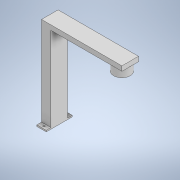
# Autodesk Inventor part: main_stand_upper_half
Saved by Autodesk Inventor 2021 (Build 250183000, 183)
## iProperties
Created: 2020-10-10
Part Number: main_stand_upper_half
Material: Generic
Document SubType Name: Modeling
Designer: bober
Density: 1 g/cm^3
Appearance: Default
Author: bober
Autodesk Inventor part; units mm, degrees
ref_plane "YZ Plane" through (0, 0, 0) normal (1, 0, 0) x (0, 1, 0)
ref_plane "XZ Plane" through (0, 0, 0) normal (0, 1, 0) x (-1, 0, 0)
ref_plane "XY Plane" through (0, 0, 0) normal (0, 0, 1) x (1, 0, 0)
sketch "Sketch1" plane through (0, 0, 0) normal (0, 1, 0) x (-1, 0, 0)
  line L0 (-10, 27.5) -> (10, 27.5)
  line L1 (10, 27.5) -> (10, -27.5)
  line L2 (10, -27.5) -> (-10, -27.5)
  line L3 (-10, -27.5) -> (-10, 27.5)
  line L4 (-10, 27.5) -> (10, -27.5) construction
  line L5 (10, 27.5) -> (-10, -27.5) construction
  point P0 (0, 0)
  dimension "d0" = 20
  dimension "d1" = 55
  constraints: 12 end point, 2 midpoint, 2 parallel, 1 horizontal, 1 perpendicular
  measures "d0" distance of L1.end L2.end
  measures "d1" distance of L0.end L1.end
extrude "Extrusion1" add sketch "Sketch1" along normal blind 3
sketch "Sketch2" plane through (0, 3, 0) normal (0, 1, 0) x (1, 0, 0)
  circle A0 centre (0, -22.5) radius 2
  circle A1 centre (0, 22.5) radius 2
  point P0 (0, 0)
  dimension "d4" = 4
  dimension "d5" = 4
  constraints: 2 centre point
  measures "d4" diameter of A0
  measures "d5" diameter of A1
extrude "Extrusion2" cut sketch "Sketch2" against normal blind 3
sketch "Sketch3" plane through (0, 3, 0) normal (0, 1, 0) x (1, 0, 0)
  line L0 (10, -17.5) -> (-10, -17.5)
  line L1 (-10, -17.5) -> (-10, 17.5)
  line L2 (-10, 17.5) -> (10, 17.5)
  line L3 (10, 17.5) -> (10, -17.5)
  line L4 (10, -17.5) -> (-10, 17.5) construction
  line L5 (-10, -17.5) -> (10, 17.5) construction
  point P0 (0, 0)
  dimension "d8" = 20
  dimension "d9" = 35
  constraints: 12 end point, 2 midpoint, 2 parallel, 1 horizontal, 1 perpendicular
  measures "d8" distance of L1.end L2.end
  measures "d9" distance of L0.end L1.end
extrude "Extrusion3" add sketch "Sketch3" along normal blind 178
sketch "Sketch4" plane through (0, 181, 0) normal (0, 1, 0) x (1, 0, 0)
  line L0 (-10, 17.5) -> (-10, -17.5) projected
  line L1 (-10, -17.5) -> (160, -17.5)
  line L2 (160, -17.5) -> (160, 17.5)
  line L3 (160, 17.5) -> (-10, 17.5)
  line L4 (-10, 17.5) -> (-10, -17.5)
  point P0 (0, 0)
  dimension "d12" = 170
  dimension "d13" = 35
  constraints: 8 end point, 2 parallel, 1 horizontal, 1 perpendicular
  measures "d12" distance of L3.end L2.end
  measures "d13" distance of L2.end L1.end
extrude "Extrusion4" add sketch "Sketch4" along normal blind 10
sketch "Sketch5" plane through (0, 181, 0) normal (0, -1, 0) x (1, 0, 0)
  circle A0 centre (142.5, 0) radius 17.5
  point P0 (0, 0)
  constraints: 1 centre point
extrude "Extrusion5" add sketch "Sketch5" along normal blind 17
body "Solid1"
